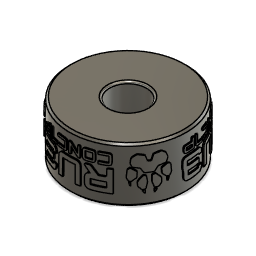
light v3 (Autodesk Fusion 360 design; units mm, degrees)
Autodesk Fusion 360 part; units mm, degrees
sketch "Esquisse1" plane through (0, 0, 0) normal (0, 1, 0) x (1, 0, 0)
  line L0 (25, 200) -> (-25, 200)
  line L1 (-25, 200) -> (-25, -200)
  line L2 (-25, -200) -> (25, -200)
  line L3 (25, -200) -> (25, 200)
  line L4 (25, 200) -> (-25, -200) construction
  line L5 (-25, 200) -> (25, -200) construction
  circle A0 centre (0, 100) radius 6.5
  circle A1 centre (0, 100) radius 4
  dimension "d1" = 50
  dimension "d2" = 400
  dimension "d3" = 13
  dimension "d4" = 8
  constraint horizontal L0
  constraint perpendicular L0 L1
  constraint parallel L0 L2
  constraint parallel L1 L3
  constraint coincident L4 origin
  constraint coincident L5 origin
  constraint concentric A0 A1
  measures "d1" distance of L1.end L2.end
  measures "d2" distance of L0.end L1.end
  measures "d3" diameter of A0
  measures "d4" diameter of A1
extrude "Extrusion1" add sketch "Esquisse1" against normal blind 6 contours L0 L1 L2 L3 makes body 1
extrude "Extrusion2" add sketch "Esquisse1" against normal blind 7 contours A0 bodies 1
fillet "Congé1" radius 3 1 edges at (-6.0601, -7, -102.3505) on bodies 1
extrude "Extrusion3" add 1 faces at (0.1619, -6, 102.1606) along direction (0, -1, 0) blind 9 and the other way blind -3 on bodies 1 bodies 1 makes body 2
extrude "Extrusion4" add sketch "Esquisse1" along normal blind -15 and the other way blind 8 contours A0 bodies 2
fillet "Congé2" radius 3 1 edges at (-6.0601, -8, -102.3505) on bodies 2
extrude "Extrusion5" add 1 faces at (0, -15, 101.3333) along direction (0, -1, 0) blind 6.5 and the other way blind -0.5 separate body on bodies 2 makes body 3
extrude "Extrusion6" add sketch "Esquisse1" along normal blind -22.5 and the other way blind 15.5 contours A0 bodies 3
fillet "Congé3" radius 3 1 edges at (-6.0601, -22.5, -102.3505) on bodies 3
extrude "Extrusion7" add sketch "Esquisse1" along normal blind 1 contours A0 bodies 1
fillet "Congé4" radius 3 1 edges at (-6.0601, 1, -97.6495) on bodies 1
extrude "Extrusion8" cut 2 faces at (-8.3333, -17.5, 200) (-8.3333, -11, 200) along direction (0, 0, -1) blind 270 on bodies 2 3 bodies 2 3
extrude "Extrusion9" add 1 faces at (-0.0996, -15, -167.9963) along direction (0, -1, 0) blind 0.25 separate body on bodies 2 makes body 4
revolve "Révolution1" add 1 faces at (-8.3333, -11, -70) angle 180 about axis through (25, -15.25, -70) along (1, 0, 0) on bodies 2 bodies 2 3 4
extrude "Extrusion10" cut 1 faces at (-0.0996, -15.25, -167.9963) along direction (0, 1, 0) blind 0.25 on bodies 2 bodies 2
sketch "Esquisse2" plane through (0, 0, 0) normal (0, -1, 0) x (1, 0, 0)
  line L0 (25, -70) -> (-25, -70)
  line L1 (-25, -70) -> (-25, -200)
  line L2 (-25, -200) -> (25, -200)
  line L3 (25, -200) -> (25, -70)
  circle A0 centre (0, -100) radius 6.5
  circle A1 centre (0, -100) radius 10
  circle A2 centre (0, -100) radius 3.5
  circle A3 centre (0, -100) radius 6.5
  line L4 (25, 200) -> (25, -200)
  line L5 (25, -200) -> (-25, -200)
  line L6 (-25, -200) -> (-25, 200)
  line L7 (-25, 200) -> (25, 200)
  dimension "d42" = 7
  constraint concentric A0 A1
  constraint concentric A1 A2
  measures "d42" diameter of A2
extrude "Extrusion11" add sketch "Esquisse2" along normal blind -1 and the other way blind 4 separate body contours A0 A3 | A1 | A2 makes body 5
fillet "Congé5" radius 2 1 edges at (-9.3233, 4, -96.3838) on bodies 5
fillet "Congé6" radius 1 1 edges at (-9.3233, 1, -96.3838) on bodies 5
extrude "Extrusion12" add sketch "Esquisse2" along normal blind 22.5 and the other way blind 1 contours A2 bodies 5
extrude "Extrusion13" add 1 faces at (1.7216, -22.5, -100.6592) along direction (0, -1, 0) blind 12 on bodies 5 bodies 5
ref_plane "Plan de construction1" through (0, 0, -100) normal (0, 0, 1) x (1, 0, 0)
sketch "Esquisse3" plane through (0, 0, -100) normal (0, 0, 1) x (1, 0, 0)
  line L0 (0, -32.5) -> (0, -22.5)
  line L1 (0, -22.5) -> (0, -22.7)
  circle A0 centre (0, -25.5) radius 1.7
  line L2 (0, -34.5) -> (-1.5, -34.5)
  line L3 (-1.5, -34.5) -> (-1.5, -32.5)
  circle A1 centre (-1.5, -32.5) radius 2
  circle A2 centre (1.5, -32.5) radius 2
  line L4 (3.5, -34.5) -> (3.5, -31.3)
  line L5 (-3.5, -34.5) -> (3.5, -34.5)
  line L6 (3.5, -34.5) -> (-3.5, -34.5)
  line L7 (-3.5, -34.5) -> (-3.5, -31.3)
  dimension "d60" = 3.4
  dimension "d65" = 1.5
  dimension "d66" = 2
  dimension "d67" = 4
  constraint vertical L0
  constraint coincident L0 L1.end
  constraint horizontal L2
  constraint perpendicular L2 L3
  constraint coincident L3.end A1.centre
  constraint symmetric L0 A1 A2
  constraint vertical L4
  constraint tangent A2 L4
  constraint coincident L4.start L5
  constraint coincident L4.start L5.end
  constraint coincident L5.start L6.end
  constraint perpendicular L6 L7
  constraint coincident L0 A0.centre
  measures "d60" diameter of A0
  measures "d65" distance of L2.start L2.end
  measures "d66" distance of L2.end L3.end
  measures "d67" diameter of A1
extrude "Extrusion14" cut sketch "Esquisse3" along normal blind 5 and the other way blind 5 contours L0 A0 | L0 A0 bodies 5
thread "Filetage2" "ISO Metric profile 7.0 M7x1 6g" major diameter 6.884 minor diameter 5.744 pitch 1 angle 60 modelled right hand crest width 0.1446 on face at (-2.0275, -19.6639, -102.8529) crest through (3.442, 1.25, -100) on bodies 5
revolve "Révolution2" cut sketch "Esquisse3" angle 360 about axis through (0, -32.5, -100) along (0, 1, 0) contours A1 L5 L6 L7 | A2 L4 L5 L6 bodies 5
sketch "Esquisse5" plane through (0, -34.5, 0) normal (0, -1, 0) x (1, 0, 0)
  circle A0 centre (0, -100) radius 1.5
  circle A1 centre (0, -100) radius 15
  circle A2 centre (0, -100) radius 3.5
  circle A3 centre (0, -100) radius 5.5
  circle A4 centre (0, -100) radius 14
  circle A5 centre (0, -100) radius 13.9
  line L0 (0, -113.9) -> (12.0378, -106.95)
  line L1 (12.0378, -106.95) -> (12.0378, -93.05)
  line L2 (12.0378, -93.05) -> (0, -86.1)
  line L3 (0, -86.1) -> (-12.0378, -93.05)
  line L4 (-12.0378, -93.05) -> (-12.0378, -106.95)
  line L5 (-12.0378, -106.95) -> (0, -113.9)
  line L6 (0, -114) -> (12.1244, -107)
  line L7 (12.1244, -107) -> (12.1244, -93)
  line L8 (12.1244, -93) -> (0, -86)
  line L9 (0, -86) -> (-12.1244, -93)
  line L10 (-12.1244, -93) -> (-12.1244, -107)
  line L11 (-12.1244, -107) -> (0, -114)
  point P0 (0, -100)
  point P1 (0, -100)
  dimension "d69" = 30
  dimension "d70" = 7
  dimension "d71" = 11
  dimension "d94" = -1
  dimension "d95" = -1.1
  constraint concentric A0 A1
  constraint concentric A1 A2
  constraint concentric A1 A3
  constraint coincident P1 P0
  constraint coincident A5 L0.start
  constraint coincident A4 L6.start
  measures "d69" diameter of A1
  measures "d70" diameter of A2
  measures "d71" diameter of A3
extrude "Extrusion16" add sketch "Esquisse5" against normal blind 7 separate body contours A2 | A3 | L0 L1 L2 L3 L4 L5 makes body 6
extrude "Extrusion19" add sketch "Esquisse5" against normal blind 7 separate body contours A0 | A1 | A2 | A3 | A4 A5 L7 | A4 A5 L8 | A5 L7 L8 | A4 A5 L6 | A5 L6 L7 | A4 A5 L9 | A5 L8 L9 | A5 L1 L7 | A5 L7 | A5 L8 | A5 L2 L8 | A5 L6 L11 | A4 A5 L11 | A5 L0 L6 | A5 L6 | A4 A5 L10 | A5 L9 L10 | A5 L9 | A5 L3 L9 | L0 L1 L2 L3 L4 L5 | A5 L10 L11 | A5 L5 L11 | A5 L11 | A5 L10 | A5 L4 L10 makes body 7
extrude "Extrusion18" add sketch "Esquisse5" along normal blind 7 contours A0 | A1 | A2 | A3 | A4 A5 L7 | A4 A5 L8 | A5 L7 L8 | A4 A5 L6 | A5 L6 L7 | A4 A5 L9 | A5 L8 L9 | A5 L1 L7 | A5 L7 | A5 L8 | A5 L2 L8 | A5 L6 L11 | A4 A5 L11 | A5 L0 L6 | A5 L6 | A4 A5 L10 | A5 L9 L10 | A5 L9 | A5 L3 L9 | L0 L1 L2 L3 L4 L5 | A5 L10 L11 | A5 L5 L11 | A5 L11 | A5 L10 | A5 L4 L10 bodies 7
chamfer "Chanfrein1" distance 0.5 angle 45 1 edges at (-13.9849, -41.5, -105.4242) on bodies 7
thread "Filetage4" "ISO Metric profile 7.0 M7x1 6H" major diameter 7.1472 minor diameter 6.0355 pitch 1 angle 60 modelled right hand crest width 0.2748 on face at (-1.3822, -29.8333, -99.4173) crest through (3.0178, -34.25, -100) on bodies 6
sketch "Esquisse8" plane through (0, -41.5, 0) normal (0, -1, 0) x (1, 0, 0)
  circle A0 centre (0, -100) radius 14.5
  line L0 (3.6323, -106.3615) -> (-0.1725, -106.3593)
  line L1 (-0.2143, -104.9499) -> (7.6688, -104.9708)
  line L2 (-0.1873, -89.7876) -> (0.9346, -89.7876)
  line L3 (-3.9773, -106.357) -> (-4.3209, -106.726)
  line L4 (-9.0437, -107.0514) -> (-9.6909, -106.1227)
  line L5 (0.9346, -89.7876) -> (1.6924, -90.8691)
  line L6 (3.9917, -98.7256) -> (1.9715, -95.3789)
  line L7 (3.1281, -92.9522) -> (3.806, -93.9537)
  line L8 (1.9715, -95.3789) -> (-0.0487, -92.0323)
  line L9 (-4.3209, -106.726) -> (-4.6645, -107.0949)
  line L10 (-8.0974, -104.9291) -> (-0.2143, -104.9499)
  line L11 (-4.1291, -98.3583) -> (-5.1879, -100.1132)
  line L12 (-6.0052, -98.5623) -> (-4.6592, -96.5217)
  line L13 (8.6765, -107.0922) -> (6.476, -107.0922)
  line L14 (4.803, -100.0724) -> (3.9917, -98.7256)
  line L15 (5.3675, -98.1557) -> (6.929, -100.5213)
  line L16 (-0.1725, -106.3593) -> (-3.9773, -106.357)
  line L17 (1.6924, -90.8691) -> (2.4502, -91.9506)
  line L18 (9.9911, -105.1511) -> (9.3338, -106.1216)
  line L19 (-7.3512, -100.603) -> (-6.0052, -98.5623)
  line L20 (3.806, -93.9537) -> (3.806, -94.8719)
  line L21 (-0.0878, -91.9667) -> (-0.127, -91.9012)
  line L22 (-0.127, -91.9012) -> (-0.1974, -91.9259)
  line L23 (7.3112, -104.2279) -> (6.8873, -103.5514)
  line L24 (2.4502, -91.9506) -> (3.1281, -92.9522)
  line L25 (-4.6645, -107.0949) -> (-6.8541, -107.0732)
  line L26 (3.806, -94.8719) -> (3.806, -95.7901)
  line L27 (-6.8541, -107.0732) -> (-9.0437, -107.0514)
  line L28 (8.46, -102.8362) -> (9.9911, -105.1511)
  line L29 (3.806, -95.7901) -> (5.3675, -98.1557)
  line L30 (-0.0487, -92.0323) -> (-0.0878, -91.9667)
  line L31 (6.476, -107.0922) -> (4.2755, -107.0922)
  line L32 (-4.1117, -94.7561) -> (-4.1117, -93.8237)
  line L33 (6.929, -100.5213) -> (8.46, -102.8362)
  line L34 (6.0639, -102.1539) -> (5.6142, -101.4192)
  line L35 (-4.1117, -95.6885) -> (-4.1117, -94.7561)
  line L36 (7.7352, -104.9044) -> (7.3112, -104.2279)
  line L37 (9.3338, -106.1216) -> (8.6765, -107.0922)
  line L38 (-5.1879, -100.1132) -> (-6.6427, -102.5212)
  line L39 (-10.3381, -105.1939) -> (-10.189, -104.9391)
  line L40 (6.8873, -103.5514) -> (6.7004, -103.2199)
  line L41 (7.702, -104.9376) -> (7.7352, -104.9044)
  line L42 (-1.669, -94.277) -> (-3.0702, -96.6033)
  line L43 (-0.1974, -91.9259) -> (-0.2678, -91.9506)
  line L44 (5.6142, -101.4192) -> (4.803, -100.0724)
  line L45 (-10.0399, -104.6843) -> (-8.6956, -102.6436)
  line L46 (-4.6592, -96.5217) -> (-4.3854, -96.1051)
  line L47 (4.2755, -107.0922) -> (3.9539, -106.7269)
  line L48 (3.9539, -106.7269) -> (3.6323, -106.3615)
  line L49 (-1.3091, -89.7876) -> (-0.1873, -89.7876)
  line L50 (7.6688, -104.9708) -> (7.702, -104.9376)
  line L51 (-3.0702, -96.6033) -> (-4.1291, -98.3583)
  line L52 (-4.3854, -96.1051) -> (-4.1117, -95.6885)
  line L53 (6.7004, -103.2199) -> (6.5135, -102.8885)
  line L54 (-2.7104, -91.8056) -> (-1.3091, -89.7876)
  line L55 (-0.2678, -91.9506) -> (-1.669, -94.277)
  line L56 (6.5135, -102.8885) -> (6.0639, -102.1539)
  line L57 (-6.6427, -102.5212) -> (-8.0974, -104.9291)
  line L58 (-8.6956, -102.6436) -> (-7.3512, -100.603)
  line L59 (-4.1117, -93.8237) -> (-2.7104, -91.8056)
  line L60 (-10.189, -104.9391) -> (-10.0399, -104.6843)
  line L61 (-9.6909, -106.1227) -> (-10.3381, -105.1939)
  line L62 (0.0438, -98.9394) -> (0.1799, -98.4652)
  line L63 (0.1799, -98.4652) -> (0.3161, -97.9909)
  line L64 (2.3261, -98.8888) -> (2.2791, -99.0929)
  line L65 (0.3615, -97.9392) -> (0.8389, -97.8251)
  line L66 (0.4669, -100.7254) -> (-0.1695, -100.7242)
  line L67 (1.398, -97.7151) -> (1.4797, -97.7192)
  line L68 (0.4669, -100.7254) -> (-0.1695, -100.7242)
  line L69 (1.7654, -97.9205) -> (2.051, -98.1218)
  line L70 (2.051, -98.1218) -> (2.1886, -98.5053)
  line L71 (2.051, -98.1218) -> (2.1886, -98.5053)
  line L72 (1.398, -97.7151) -> (1.4797, -97.7192)
  line L73 (2.3261, -98.8888) -> (2.2791, -99.0929)
  line L74 (0.3388, -97.9651) -> (0.3615, -97.9392)
  line L75 (0.7858, -103.6458) -> (0.6253, -103.8385)
  line L76 (0.8389, -97.8251) -> (1.3164, -97.7111)
  line L77 (0.4621, -103.766) -> (0.4593, -103.5007)
  line L78 (-0.604, -101.2643) -> (-0.5379, -101.7499)
  line L79 (0.4648, -104.0313) -> (0.4621, -103.766)
  line L80 (0.3615, -97.9392) -> (0.8389, -97.8251)
  line L81 (-2.2222, -101.657) -> (-2.5922, -101.957)
  line L82 (2.7983, -100.7801) -> (2.8481, -101.4264)
  line L83 (2.2791, -99.0929) -> (2.2322, -99.297)
  line L84 (-2.4384, -99.6984) -> (-2.5818, -99.4161)
  line L85 (2.1886, -98.5053) -> (2.3261, -98.8888)
  line L86 (1.8369, -101.6417) -> (1.5066, -101.3336)
  line L87 (0.1328, -101.7824) -> (0.1328, -101.2414)
  line L88 (-0.6144, -98.4472) -> (-0.4648, -98.8888)
  line L89 (0.1799, -98.4652) -> (0.3161, -97.9909)
  line L90 (0.6253, -103.8385) -> (0.4648, -104.0313)
  line L91 (0.0438, -98.9394) -> (0.1799, -98.4652)
  line L92 (-2.4384, -99.6984) -> (-2.5818, -99.4161)
  line L93 (-0.2105, -98.9141) -> (0.0438, -98.9394)
  line L94 (2.1886, -98.5053) -> (2.3261, -98.8888)
  line L95 (2.2791, -99.0929) -> (2.2322, -99.297)
  line L96 (-2.9199, -101.909) -> (-3.0739, -101.6445)
  line L97 (1.7654, -97.9205) -> (2.051, -98.1218)
  line L98 (-1.057, -101.1335) -> (-0.9314, -101.1348)
  line L99 (-0.764, -98.0056) -> (-0.6144, -98.4472)
  line L100 (-1.4182, -99.9122) -> (-1.6018, -99.8695)
  line L101 (1.4797, -97.7192) -> (1.7654, -97.9205)
  line L102 (-1.8307, -97.7061) -> (-1.3304, -97.8228)
  line L103 (-2.4722, -98.111) -> (-2.1515, -97.9085)
  line L104 (-1.4182, -99.9122) -> (-1.6018, -99.8695)
  line L105 (1.3164, -97.7111) -> (1.398, -97.7151)
  line L106 (-0.8301, -97.9395) -> (-0.797, -97.9726)
  line L107 (-0.5632, -102.6892) -> (-0.6544, -103.1429)
  line L108 (-2.6424, -102.113) -> (-2.6424, -102.4151)
  line L109 (-0.6144, -98.4472) -> (-0.4648, -98.8888)
  line L110 (1.4797, -97.7192) -> (1.7654, -97.9205)
  line L111 (0.3161, -97.9909) -> (0.3388, -97.9651)
  line L112 (-0.4648, -98.8888) -> (-0.2105, -98.9141)
  line L113 (0.3161, -97.9909) -> (0.3388, -97.9651)
  line L114 (-2.6849, -98.7835) -> (-2.6447, -98.4333)
  line L115 (1.3164, -97.7111) -> (1.398, -97.7151)
  line L116 (-0.4648, -98.8888) -> (-0.2105, -98.9141)
  line L117 (0.8389, -97.8251) -> (1.3164, -97.7111)
  line L118 (0.3388, -97.9651) -> (0.3615, -97.9392)
  line L119 (0.5989, -101.0519) -> (1.0189, -101.496)
  line L120 (-1.636, -101.8274) -> (-1.3465, -101.4804)
  line L121 (-0.797, -97.9726) -> (-0.764, -98.0056)
  line L122 (-1.8307, -97.7061) -> (-1.3304, -97.8228)
  line L123 (-0.797, -97.9726) -> (-0.764, -98.0056)
  line L124 (-2.7252, -99.1337) -> (-2.6849, -98.7835)
  line L125 (-0.8059, -100.7229) -> (-0.8957, -100.6629)
  line L126 (-2.905, -102.113) -> (-2.7737, -102.113)
  line L127 (0.8675, -100.0614) -> (0.745, -100.2178)
  line L128 (0.5487, -101.0519) -> (0.5738, -101.0519)
  line L129 (-3.1118, -100.1414) -> (-2.9434, -99.9845)
  line L130 (2.1672, -101.9498) -> (1.8369, -101.6417)
  line L131 (-1.7749, -102.4757) -> (-1.8038, -102.1539)
  line L132 (0.6226, -103.5007) -> (0.7858, -103.5007)
  line L133 (0.9899, -99.9051) -> (0.8675, -100.0614)
  line L134 (-2.7561, -101.933) -> (-2.9199, -101.909)
  line L135 (0.745, -100.2178) -> (0.606, -100.4716)
  line L136 (1.5066, -101.3336) -> (1.4727, -100.8867)
  line L137 (0.3407, -101.1466) -> (0.5487, -101.0519)
  line L138 (-2.7183, -102.6395) -> (-2.7941, -102.562)
  line L139 (2.3884, -102.1106) -> (2.2571, -102.1106)
  line L140 (2.2571, -102.1106) -> (2.2571, -102.4126)
  line L141 (2.8481, -101.4264) -> (2.7128, -101.6881)
  line L142 (-1.8354, -100.8921) -> (-1.8522, -101.3569)
  line L143 (1.4727, -100.8867) -> (1.4388, -100.4397)
  line L144 (1.2219, -102.9797) -> (1.005, -103.2641)
  line L145 (-2.247, -100.1274) -> (-1.8186, -100.4273)
  line L146 (-1.7854, -99.8268) -> (-2.1119, -99.7626)
  line L147 (2.7128, -101.6881) -> (2.5774, -101.9498)
  line L148 (1.4389, -101.94) -> (1.4389, -102.3177)
  line L149 (0.1328, -101.2414) -> (0.3407, -101.1466)
  line L150 (-1.8522, -101.3569) -> (-2.2222, -101.657)
  line L151 (-0.1695, -100.7242) -> (-0.8059, -100.7229)
  line L152 (2.0221, -99.7149) -> (1.506, -99.81)
  line L153 (-0.9987, -103.3374) -> (-1.2228, -103.3374)
  line L154 (0.606, -100.4716) -> (0.4669, -100.7254)
  line L155 (2.6038, -100.0241) -> (2.7484, -100.1338)
  line L156 (2.4088, -102.5596) -> (2.4642, -102.3351)
  line L157 (-1.2018, -100.2576) -> (-1.4182, -99.9122)
  line L158 (-1.8186, -100.4273) -> (-1.8354, -100.8921)
  line L159 (1.4389, -102.3177) -> (1.4389, -102.6953)
  line L160 (-2.8496, -102.3375) -> (-2.905, -102.113)
  line L161 (-2.6424, -102.7171) -> (-2.7183, -102.6395)
  line L162 (2.2571, -102.7146) -> (2.3329, -102.6371)
  line L163 (0.8675, -100.0614) -> (0.745, -100.2178)
  line L164 (1.8461, -100.1744) -> (2.2534, -99.9092)
  line L165 (2.7484, -100.1338) -> (2.7983, -100.7801)
  line L166 (-0.765, -103.4191) -> (-0.765, -103.7047)
  line L167 (-1.0035, -103.495) -> (-0.8875, -103.4216)
  line L168 (-2.7749, -99.8275) -> (-2.7252, -99.8275)
  line L169 (-0.7146, -103.2402) -> (-0.7747, -103.3374)
  line L170 (-3.2279, -101.38) -> (-3.1699, -100.7607)
  line L171 (-0.9812, -103.7794) -> (-1.1195, -103.5684)
  line L172 (-0.7747, -103.3374) -> (-0.9987, -103.3374)
  line L173 (-1.7854, -99.8268) -> (-2.1119, -99.7626)
  line L174 (0.4458, -103.215) -> (0.2893, -102.7692)
  line L175 (2.0221, -99.7149) -> (1.506, -99.81)
  line L176 (-1.2228, -103.3374) -> (-1.4844, -103.0675)
  line L177 (0.2893, -102.7692) -> (0.1328, -102.3234)
  line L178 (-2.7252, -99.8275) -> (-2.6755, -99.8275)
  line L179 (2.4642, -102.3351) -> (2.5197, -102.1106)
  line L180 (-0.8263, -103.4203) -> (-0.765, -103.4191)
  line L181 (0.7858, -103.5733) -> (0.7858, -103.6458)
  line L182 (-1.6018, -99.8695) -> (-1.7854, -99.8268)
  line L183 (1.005, -103.2641) -> (0.7254, -103.2396)
  line L184 (0.4593, -103.5007) -> (0.6226, -103.5007)
  line L185 (-0.6544, -103.1429) -> (-0.7146, -103.2402)
  line L186 (-1.1195, -103.5684) -> (-1.0035, -103.495)
  line L187 (2.3563, -99.9118) -> (2.4592, -99.9143)
  line L188 (-3.0739, -101.6445) -> (-3.2279, -101.38)
  line L189 (-0.765, -103.7047) -> (-0.765, -103.9904)
  line L190 (-0.804, -103.9904) -> (-0.8429, -103.9904)
  line L191 (-0.765, -103.9904) -> (-0.804, -103.9904)
  line L192 (-0.8875, -103.4216) -> (-0.8263, -103.4203)
  line L193 (-0.8429, -103.9904) -> (-0.9812, -103.7794)
  line L194 (2.5774, -101.9498) -> (2.3723, -101.9498)
  line L195 (0.7858, -103.5007) -> (0.7858, -103.5733)
  line L196 (-2.1119, -99.7626) -> (-2.4384, -99.6984)
  line L197 (2.2571, -102.4126) -> (2.2571, -102.7146)
  line L198 (0.745, -100.2178) -> (0.606, -100.4716)
  line L199 (-0.8957, -100.6629) -> (-0.9855, -100.603)
  line L200 (-1.3465, -101.4804) -> (-1.057, -101.1335)
  line L201 (0.606, -100.4716) -> (0.4669, -100.7254)
  line L202 (1.4388, -100.4397) -> (1.8461, -100.1744)
  line L203 (-2.5818, -99.4161) -> (-2.7252, -99.1337)
  line L204 (-0.9855, -100.603) -> (-1.2018, -100.2576)
  line L205 (-1.6018, -99.8695) -> (-1.7854, -99.8268)
  line L206 (-2.1515, -97.9085) -> (-1.8307, -97.7061)
  line L207 (2.4592, -99.9143) -> (2.6038, -100.0241)
  line L208 (-2.6447, -98.4333) -> (-2.5584, -98.2721)
  line L209 (2.3723, -101.9498) -> (2.1672, -101.9498)
  line L210 (-2.1119, -99.7626) -> (-2.4384, -99.6984)
  line L211 (-0.8059, -100.7229) -> (-0.8957, -100.6629)
  line L212 (-2.5584, -98.2721) -> (-2.4722, -98.111)
  line L213 (0.9899, -99.9051) -> (0.8675, -100.0614)
  line L214 (1.4389, -102.6953) -> (1.2219, -102.9797)
  line L215 (0.5738, -101.0519) -> (0.5989, -101.0519)
  line L216 (2.1271, -99.5059) -> (2.0221, -99.7149)
  line L217 (-2.7941, -102.562) -> (-2.8496, -102.3375)
  line L218 (-2.5818, -99.4161) -> (-2.7252, -99.1337)
  line L219 (-2.5922, -101.957) -> (-2.7561, -101.933)
  line L220 (-0.5379, -101.7499) -> (-0.4719, -102.2355)
  line L221 (-3.1699, -100.7607) -> (-3.1118, -100.1414)
  line L222 (2.3329, -102.6371) -> (2.4088, -102.5596)
  line L223 (2.2322, -99.297) -> (2.1271, -99.5059)
  line L224 (-0.1695, -100.7242) -> (-0.8059, -100.7229)
  line L225 (-2.6447, -98.4333) -> (-2.5584, -98.2721)
  line L226 (-1.8038, -102.1539) -> (-1.7199, -101.9906)
  line L227 (-1.2018, -100.2576) -> (-1.4182, -99.9122)
  line L228 (-0.764, -98.0056) -> (-0.6144, -98.4472)
  line L229 (-2.6849, -98.7835) -> (-2.6447, -98.4333)
  line L230 (-0.2105, -98.9141) -> (0.0438, -98.9394)
  line L231 (1.0189, -101.496) -> (1.4389, -101.94)
  line L232 (2.2322, -99.297) -> (2.1271, -99.5059)
  line L233 (-2.6424, -102.4151) -> (-2.6424, -102.7171)
  line L234 (-2.4722, -98.111) -> (-2.1515, -97.9085)
  line L235 (-2.7737, -102.113) -> (-2.6424, -102.113)
  line L236 (-0.7049, -101.2002) -> (-0.604, -101.2643)
  line L237 (-1.3304, -97.8228) -> (-0.8301, -97.9395)
  line L238 (-2.5584, -98.2721) -> (-2.4722, -98.111)
  line L239 (0.1328, -102.3234) -> (0.1328, -101.7824)
  line L240 (-0.8301, -97.9395) -> (-0.797, -97.9726)
  line L241 (-2.9434, -99.9845) -> (-2.7749, -99.8275)
  line L242 (2.1271, -99.5059) -> (2.0221, -99.7149)
  line L243 (-1.3304, -97.8228) -> (-0.8301, -97.9395)
  line L244 (-0.9314, -101.1348) -> (-0.8059, -101.136)
  line L245 (-0.8059, -101.136) -> (-0.7049, -101.2002)
  line L246 (2.2534, -99.9092) -> (2.3563, -99.9118)
  line L247 (-1.746, -102.7976) -> (-1.7749, -102.4757)
  line L248 (1.506, -99.81) -> (0.9899, -99.9051)
  line L249 (-0.9855, -100.603) -> (-1.2018, -100.2576)
  line L250 (-0.4719, -102.2355) -> (-0.5632, -102.6892)
  line L251 (0.7254, -103.2396) -> (0.4458, -103.215)
  line L252 (-1.7199, -101.9906) -> (-1.636, -101.8274)
  line L253 (2.5197, -102.1106) -> (2.3884, -102.1106)
  line L254 (-0.8957, -100.6629) -> (-0.9855, -100.603)
  line L255 (-2.7252, -99.1337) -> (-2.6849, -98.7835)
  line L256 (-2.6755, -99.8275) -> (-2.247, -100.1274)
  line L257 (-1.4844, -103.0675) -> (-1.746, -102.7976)
  line L258 (1.506, -99.81) -> (0.9899, -99.9051)
  line L259 (-2.1515, -97.9085) -> (-1.8307, -97.7061)
  circle A1 centre (0, -100) radius 14.5
emboss "Gravure en relief2" depth -0.4 profiles "Esquisse8" section 1 contours L0 L2 L3 L4 L5 L7 L9 L12 L13 L15 L16 L17 L18 L19 L20 L24 L25 L26 L27 L28 L29 L31 L32 L33 L35 L37 L39 L45 L46 L47 L48 L49 L52 L54 L58 L59 L60 L61 | L62 L63 L64 L65 L66 L67 L68 L69 L70 L71 L72 L73 L74 L76 L80 L83 L84 L85 L88 L89 L91 L92 L93 L94 L95 L97 L99 L100 L101 L102 L103 L104 L105 L106 L109 L110 L111 L112 L113 L114 L115 L116 L117 L118 L121 L122 L123 L124 L125 L127 L133 L135 L146 L151 L152 L154 L157 L163 L173 L175 L182 L196 L198 L199 L201 L203 L204 L205 L206 L208 L210 L211 L212 L213 L216 L218 L223 L224 L225 L227 L228 L229 L230 L232 L234 L237 L238 L240 L242 L243 L248 L249 L254 L255 L258 L259 | L75 L77 L79 L90 L132 L181 L184 L195 | L78 L98 L107 L120 L131 L153 L169 L172 L176 L185 L200 L220 L226 L236 L244 L245 L247 L250 L252 L257 | L81 L96 L129 L134 L142 L145 L150 L158 L168 L170 L178 L188 L219 L221 L241 L256 | L82 L86 L130 L136 L141 L143 L147 L155 L164 L165 L187 L194 L202 L207 L209 L246 | L87 L119 L128 L137 L144 L148 L149 L159 L174 L177 L183 L214 L215 L231 L239 L251 | L108 L126 L138 L160 L161 L217 L233 L235 | L139 L140 L156 L162 L179 L197 L222 L253 | L166 L167 L171 L180 L186 L189 L190 L191 L192 L193 onto face at (9.3024, -41.5, -103.9344) on bodies 7 bodies 7
sketch "Esquisse9" plane through (0, 0, 0) normal (0, 0, 1) x (1, 0, 0)
  line L0 (18.0757, -34.7535) -> (18.0282, -34.1284)
  line L1 (11.4541, -34.8184) -> (11.5353, -33.9522)
  line L2 (13.4251, -33.4859) -> (13.4016, -34.136)
  line L3 (14.4903, -34.4736) -> (14.6659, -34.4754)
  line L4 (19.8821, -33.9793) -> (19.9518, -34.8832)
  line L5 (-7.8492, -34.7645) -> (-7.8492, -35.2972)
  spline S0 degree 3 poles (7.4266, -29.6855) (8.5421, -29.6855) (8.5702, -29.6892) (8.7408, -29.8598) knots 0 0 0 0 1 1 1 1
  line L6 (-7.5083, -30.5933) -> (-6.6061, -30.5734)
  line L7 (-6.2864, -34.2317) -> (-7.8492, -34.2317)
  line L8 (1.1658, -31.2181) -> (0.6395, -30.5841)
  line L9 (0.0357, -32.3934) -> (0.0357, -31.0394)
  line L10 (-8.1195, -31.4791) -> (-8.1411, -31.8165)
  line L11 (-6.6061, -30.5734) -> (-6.5849, -30.1294)
  line L12 (3.7296, -31.0351) -> (3.7296, -31.8165)
  spline S1 degree 3 poles (-8.5303, -32.15) (-8.7648, -31.8771) (-8.7799, -31.0828) (-8.556, -30.7982) knots 0 0 0 0 1 1 1 1
  line L13 (-5.2564, -29.6855) -> (-5.0078, -29.6855)
  line L14 (-3.0898, -32.1054) -> (-3.0898, -31.8165)
  spline S2 degree 3 poles (5.7352, -29.928) (5.7639, -29.9704) (5.7879, -30.4717) (5.7885, -31.0419) knots 0 0 0 0 1 1 1 1
  line L15 (-8.359, -32.3493) -> (-8.5303, -32.15)
  line L16 (-6.2815, -29.6855) -> (-5.9991, -29.6855)
  line L17 (0.604, -31.4667) -> (0.5685, -32.3493)
  line L18 (-1.6002, -38.5648) -> (-2.1701, -38.5648)
  line L19 (-4.5105, -35.8655) -> (-4.5105, -36.4338)
  spline S3 degree 3 poles (-4.2168, -32.3848) (-5.0338, -32.3848) (-5.1505, -32.3692) (-5.3179, -32.2376) knots 0 0 0 0 1 1 1 1
  line L20 (-5.505, -29.6855) -> (-5.2564, -29.6855)
  line L21 (5.2924, -31.0351) -> (5.2924, -30.2537)
  line L22 (8.3469, -31.8165) -> (8.3469, -31.0351)
  spline S4 degree 3 poles (5.7885, -31.0419) (5.7899, -32.3794) (5.824, -32.34) (4.6394, -32.3731) knots 0 0 0 0 1 1 1 1
  line L23 (7.3169, -31.8165) -> (8.3469, -31.8165)
  line L24 (-8.1411, -31.8165) -> (-7.3558, -31.8165)
  line L25 (-7.8492, -35.2972) -> (-6.1799, -35.2972)
  line L26 (-2.7401, -38.5648) -> (-2.7196, -36.1903)
  line L27 (-4.1554, -37.0021) -> (-3.5871, -37.0021)
  line L28 (-7.6361, -36.931) -> (-7.6361, -37.4283)
  line L29 (-3.981, -38.2839) -> (-4.2341, -38.5293)
  line L30 (-4.7236, -37.4283) -> (-4.7236, -37.2152)
  spline S5 degree 3 poles (8.7408, -29.8598) (8.9093, -30.0283) (8.9151, -30.067) (8.9129, -31.0141) knots 0 0 0 0 1 1 1 1
  line L31 (0.3021, -32.3713) -> (0.0357, -32.3934)
  spline S6 degree 3 poles (-8.556, -30.7982) (-8.4146, -30.6183) (-8.385, -30.6126) (-7.5083, -30.5933) knots 0 0 0 0 1 1 1 1
  line L32 (6.2869, -31.8165) -> (7.3169, -31.8165)
  line L33 (9.1283, -38.5648) -> (6.7591, -38.5648)
  spline S7 degree 3 poles (-0.6487, -29.8327) (-0.4616, -29.9799) (-0.4615, -29.9802) (-0.4615, -31.0293) knots 0 0 0 0 1 1 1 1
  line L34 (-3.0898, -29.9696) -> (-3.0898, -29.6855)
  line L35 (-3.3029, -32.1007) -> (-3.3029, -32.3848)
  line L36 (-7.6361, -37.4283) -> (-6.1799, -37.4283)
  line L37 (-7.3342, -31.1215) -> (-8.0978, -31.1417)
  line L38 (-6.5638, -29.6855) -> (-6.2815, -29.6855)
  spline S8 degree 3 poles (-8.7725, -36.9242) (-8.7727, -36.2516) (-8.8006, -35.9736) (-8.8849, -35.8045) knots 0 0 0 0 1 1 1 1
  line L39 (-3.5871, -37.0021) -> (-3.5875, -37.2685)
  line L40 (-2.1701, -38.5648) -> (-2.7401, -38.5648)
  spline S9 degree 3 poles (-8.2584, -38.425) (-8.6945, -38.1556) (-8.7722, -37.929) (-8.7725, -36.9242) knots 0 0 0 0 1 1 1 1
  spline S10 degree 3 poles (-8.8032, -33.544) (-8.4911, -33.1191) (-8.3574, -33.0954) (-6.2792, -33.0952) knots 0 0 0 0 1 1 1 1
  line L41 (6.3579, -36.0786) -> (4.7951, -36.0786)
  line L42 (-5.0078, -29.6855) -> (-5.0078, -30.751)
  line L43 (-3.0898, -30.2537) -> (-3.0898, -29.9696)
  line L44 (-6.5849, -30.1294) -> (-6.5638, -29.6855)
  line L45 (6.3605, -34.942) -> (7.1073, -34.942)
  line L46 (-6.5706, -31.4589) -> (-6.5706, -31.1014)
  line L47 (-5.3179, -32.2376) -> (-5.505, -32.0903)
  line L48 (5.2924, -31.8165) -> (5.2924, -31.0351)
  line L49 (2.1512, -30.5897) -> (2.171, -29.6855)
  line L50 (-1.5814, -36.416) -> (-1.6002, -38.5648)
  spline S11 degree 3 poles (2.4298, -32.3848) (2.1652, -32.3848) (2.0329, -32.2627) (1.1658, -31.2181) knots 0 0 0 0 1 1 1 1
  line L51 (7.9562, -33.1306) -> (8.5422, -33.11)
  line L52 (-7.1984, -32.3493) -> (-8.359, -32.3493)
  spline S12 degree 3 poles (7.1073, -34.942) (7.6895, -34.942) (7.8627, -34.9196) (7.8931, -34.8404) knots 0 0 0 0 1 1 1 1
  line L53 (5.2924, -30.2537) -> (4.511, -30.2537)
  line L54 (4.7951, -37.4283) -> (6.3579, -37.4283)
  line L55 (-5.505, -32.0903) -> (-5.505, -30.8879)
  line L56 (6.2869, -32.1007) -> (6.2869, -31.8165)
  spline S13 degree 3 poles (5.541, -29.7703) (5.6191, -29.8147) (5.7065, -29.8856) (5.7352, -29.928) knots 0 0 0 0 1 1 1 1
  line L57 (-6.0185, -31.0174) -> (-6.0378, -32.3493)
  line L58 (-3.0898, -32.3944) -> (-3.0898, -32.1054)
  line L59 (6.2869, -29.9696) -> (6.2869, -29.6855)
  line L60 (0.5685, -32.3493) -> (0.3021, -32.3713)
  line L61 (6.2869, -30.2537) -> (6.2869, -29.9696)
  spline S14 degree 3 poles (0.3144, -29.6855) (0.5837, -29.6855) (0.6188, -29.7158) (1.3622, -30.5897) knots 0 0 0 0 1 1 1 1
  spline S15 degree 3 poles (8.9129, -31.0141) (8.9097, -32.3864) (8.9115, -32.3848) (7.3571, -32.3848) knots 0 0 0 0 1 1 1 1
  spline S16 degree 3 poles (-8.9737, -34.662) (-8.9535, -33.868) (-8.9305, -33.7173) (-8.8032, -33.544) knots 0 0 0 0 1 1 1 1
  line L62 (7.3169, -30.2537) -> (6.2869, -30.2537)
  line L63 (7.3571, -32.3848) -> (6.2869, -32.3848)
  line L64 (0.0357, -31.0394) -> (0.0357, -29.6855)
  line L65 (8.3469, -30.2537) -> (7.3169, -30.2537)
  line L66 (6.2869, -32.3848) -> (6.2869, -32.1007)
  line L67 (0.0357, -29.6855) -> (0.3144, -29.6855)
  line L68 (8.3469, -31.0351) -> (8.3469, -30.2537)
  line L69 (0.6395, -30.5841) -> (0.604, -31.4667)
  line L70 (-0.9588, -31.0351) -> (-0.9588, -30.2537)
  line L71 (18.5504, -33.1323) -> (19.12, -32.7612)
  line L72 (7.9441, -33.9347) -> (7.9562, -33.1306)
  spline S17 degree 3 poles (7.9295, -36.8955) (7.9295, -36.6806) (7.9275, -36.4089) (7.9251, -36.2917) knots 0 0 0 0 1 1 1 1
  line L73 (14.8539, -30.0528) -> (14.9001, -30.099)
  line L74 (16.3732, -36.7612) -> (16.1543, -36.1377)
  line L75 (-3.3029, -32.3848) -> (-4.2168, -32.3848)
  spline S18 degree 3 poles (6.3579, -37.4283) (7.3494, -37.4283) (7.9223, -37.4023) (7.9251, -37.3572) knots 0 0 0 0 1 1 1 1
  line L76 (16.8161, -33.5478) -> (16.6216, -33.9028)
  line L77 (19.3374, -36.468) -> (19.4149, -36.1541)
  line L78 (17.0696, -37.9849) -> (16.8431, -38.2568)
  line L79 (12.3578, -32.0716) -> (12.1572, -31.6767)
  line L80 (-2.0243, -30.2537) -> (-3.0898, -30.2537)
  line L81 (7.9207, -36.0786) -> (6.3579, -36.0786)
  line L82 (19.2217, -31.3343) -> (19.1561, -31.6197)
  spline S19 degree 3 poles (4.4545, -29.6876) (5.0236, -29.6889) (5.4554, -29.7218) (5.541, -29.7703) knots 0 0 0 0 1 1 1 1
  line L83 (17.0105, -33.1929) -> (16.8161, -33.5478)
  line L84 (19.1252, -35.8401) -> (19.1252, -36.2625)
  line L85 (-3.5672, -34.5869) -> (-4.1454, -34.5869)
  line L86 (3.7296, -31.8165) -> (4.511, -31.8165)
  line L87 (14.1079, -29.8434) -> (14.8076, -30.0066)
  line L88 (18.9435, -32.1973) -> (18.7966, -32.4895)
  line L89 (17.8096, -29.6871) -> (17.9238, -29.6928)
  line L90 (16.592, -37.3847) -> (16.3732, -36.7612)
  line L91 (13.4716, -32.6461) -> (13.015, -32.5563)
  line L92 (13.7284, -32.7058) -> (13.4716, -32.6461)
  line L93 (12.5111, -30.2464) -> (12.9596, -29.9633)
  line L94 (19.1252, -36.2625) -> (19.1252, -36.6849)
  line L95 (19.0294, -30.7979) -> (19.2217, -31.3343)
  line L96 (-0.9588, -31.8165) -> (-0.9588, -31.0351)
  line L97 (19.8124, -33.0754) -> (19.8821, -33.9793)
  line L98 (-3.3029, -31.8165) -> (-3.3029, -32.1007)
  spline S20 degree 3 poles (7.9251, -37.3572) (7.9275, -37.3182) (7.9295, -37.1104) (7.9295, -36.8955) knots 0 0 0 0 1 1 1 1
  line L99 (-4.7236, -34.2317) -> (-6.2864, -34.2317)
  line L100 (19.0904, -31.905) -> (18.9435, -32.1973)
  spline S21 degree 3 poles (-1.9628, -29.6855) (-0.9303, -29.6855) (-0.8202, -29.6978) (-0.6487, -29.8327) knots 0 0 0 0 1 1 1 1
  line L101 (17.9238, -29.6928) -> (18.038, -29.6985)
  line L102 (19.1252, -36.6849) -> (19.2313, -36.5765)
  line L103 (5.5985, -34.0186) -> (6.3605, -34.942)
  line L104 (14.7159, -33.8155) -> (14.5902, -33.7316)
  line L105 (12.5583, -32.4665) -> (12.3578, -32.0716)
  line L106 (-3.6089, -34.1826) -> (-3.5672, -34.5869)
  line L107 (-6.1799, -37.4283) -> (-4.7236, -37.4283)
  line L108 (-4.2341, -38.5293) -> (-6.1305, -38.5487)
  line L109 (11.5353, -33.9522) -> (11.6165, -33.0861)
  line L110 (19.6101, -32.922) -> (19.8124, -33.0754)
  line L111 (16.2202, -30.7418) -> (16.4106, -30.0785)
  line L112 (-3.0898, -31.8165) -> (-2.0243, -31.8165)
  spline S22 degree 3 poles (-4.1546, -33.255) (-3.7949, -33.4998) (-3.6548, -33.738) (-3.6089, -34.1826) knots 0 0 0 0 1 1 1 1
  line L113 (12.1572, -32.6471) -> (12.2268, -32.6471)
  line L114 (13.015, -32.5563) -> (12.5583, -32.4665)
  line L115 (-6.0378, -32.3493) -> (-7.1984, -32.3493)
  spline S23 degree 3 poles (3.3016, -32.1699) (3.1752, -32.0435) (3.1613, -31.9306) (3.1613, -31.0319) knots 0 0 0 0 1 1 1 1
  line L116 (18.4375, -29.98) -> (18.8371, -30.2615)
  line L117 (19.2313, -36.5765) -> (19.3374, -36.468)
  spline S24 degree 3 poles (3.1613, -31.0319) (3.1613, -30.0673) (3.1671, -30.0284) (3.3357, -29.8598) knots 0 0 0 0 1 1 1 1
  line L118 (-3.0898, -29.6855) -> (-1.9628, -29.6855)
  line L119 (16.8431, -38.2568) -> (16.6186, -38.5263)
  line L120 (16.0298, -31.405) -> (16.2202, -30.7418)
  line L121 (-7.3558, -31.8165) -> (-6.5706, -31.8165)
  line L122 (16.6186, -38.5263) -> (16.6148, -38.1552)
  line L123 (17.9809, -36.6579) -> (17.6775, -37.0556)
  spline S25 degree 3 poles (-2.7196, -36.1903) (-2.6999, -33.9089) (-2.6933, -33.8078) (-2.5505, -33.6152) knots 0 0 0 0 1 1 1 1
  line L124 (-4.7236, -37.0021) -> (-4.1554, -37.0021)
  line L125 (17.6775, -37.0556) -> (17.3741, -37.4534)
  line L126 (17.1419, -29.8466) -> (17.8096, -29.6871)
  line L127 (3.7296, -30.2537) -> (3.7296, -31.0351)
  line L128 (17.3741, -37.4534) -> (16.9831, -37.419)
  line L129 (-8.0978, -31.1417) -> (-8.1195, -31.4791)
  line L130 (9.1283, -35.8271) -> (9.1283, -38.5648)
  line L131 (17.0676, -37.8857) -> (17.0696, -37.9849)
  line L132 (-4.1554, -31.8165) -> (-3.3029, -31.8165)
  line L133 (16.4423, -30.0423) -> (16.4741, -30.0061)
  line L134 (19.12, -32.7612) -> (19.2639, -32.7649)
  spline S26 degree 3 poles (3.3357, -29.8598) (3.5035, -29.6919) (3.545, -29.6855) (4.4545, -29.6876) knots 0 0 0 0 1 1 1 1
  line L135 (-5.9991, -29.6855) -> (-6.0185, -31.0174)
  spline S27 degree 3 poles (7.8931, -34.8404) (7.9145, -34.7845) (7.9375, -34.3769) (7.9441, -33.9347) knots 0 0 0 0 1 1 1 1
  line L136 (17.353, -32.7556) -> (17.1818, -32.9742)
  line L137 (2.171, -29.6855) -> (2.4175, -29.6855)
  line L138 (-5.505, -30.8879) -> (-5.505, -29.6855)
  line L139 (-7.8492, -34.2317) -> (-7.8492, -34.7645)
  line L140 (2.664, -32.3848) -> (2.4298, -32.3848)
  line L141 (16.6148, -38.1552) -> (16.611, -37.7842)
  line L142 (16.6216, -33.9028) -> (15.7316, -33.9011)
  line L143 (-1.5626, -34.2672) -> (-1.5814, -36.416)
  line L144 (16.611, -37.7842) -> (16.8393, -37.7842)
  line L145 (-1.925, -32.3718) -> (-3.0898, -32.3944)
  line L146 (17.9808, -33.5033) -> (18.5504, -33.1323)
  line L147 (16.9831, -37.419) -> (16.592, -37.3847)
  line L148 (-7.6361, -36.4338) -> (-7.6361, -36.931)
  spline S28 degree 3 poles (-0.4615, -31.0293) (-0.4615, -32.4182) (-0.3783, -32.3419) (-1.925, -32.3718) knots 0 0 0 0 1 1 1 1
  line L149 (-4.7236, -37.2152) -> (-4.7236, -37.0021)
  line L150 (-6.0733, -36.4338) -> (-7.6361, -36.4338)
  spline S29 degree 3 poles (-8.8849, -35.8045) (-8.974, -35.6259) (-8.9923, -35.391) (-8.9737, -34.662) knots 0 0 0 0 1 1 1 1
  spline S30 degree 3 poles (-6.1305, -38.5487) (-7.9254, -38.5669) (-8.0392, -38.5603) (-8.2584, -38.425) knots 0 0 0 0 1 1 1 1
  line L151 (9.1283, -33.0894) -> (9.1283, -35.8271)
  line L152 (-0.9588, -30.2537) -> (-2.0243, -30.2537)
  line L153 (16.8393, -37.7842) -> (17.0676, -37.7842)
  line L154 (6.2869, -29.6855) -> (7.4266, -29.6855)
  line L155 (16.4106, -30.0785) -> (16.4423, -30.0423)
  line L156 (8.5422, -33.11) -> (9.1283, -33.0894)
  line L157 (-6.5706, -31.8165) -> (-6.5706, -31.4589)
  line L158 (17.0676, -37.7842) -> (17.0676, -37.8857)
  line L159 (4.8365, -33.0951) -> (5.5985, -34.0186)
  line L160 (-6.5706, -31.1014) -> (-7.3342, -31.1215)
  spline S31 degree 3 poles (-3.5875, -37.2685) (-3.5882, -37.7033) (-3.7121, -38.0231) (-3.981, -38.2839) knots 0 0 0 0 1 1 1 1
  line L161 (18.0748, -32.6226) -> (17.353, -32.7556)
  line L162 (19.2639, -32.7649) -> (19.4079, -32.7685)
  line L163 (7.9251, -36.2917) -> (7.9207, -36.0786)
  line L164 (19.1561, -31.6197) -> (19.0904, -31.905)
  line L165 (2.1313, -31.4939) -> (2.1512, -30.5897)
  line L166 (-5.0078, -30.751) -> (-5.0078, -31.8165)
  line L167 (4.511, -31.8165) -> (5.2924, -31.8165)
  line L168 (2.664, -29.6855) -> (2.664, -31.0351)
  line L169 (13.4016, -34.136) -> (13.3781, -34.786)
  line L170 (14.0854, -34.9588) -> (14.4903, -34.4736)
  line L171 (14.9827, -34.5668) -> (15.1239, -34.6565)
  line L172 (11.9057, -35.8435) -> (12.0893, -35.8435)
  line L173 (13.5631, -35.6723) -> (13.6805, -35.444)
  line L174 (13.3781, -34.786) -> (12.8606, -35.2057)
  line L175 (11.6695, -35.1882) -> (11.4541, -34.8184)
  line L176 (11.9832, -36.1575) -> (11.9057, -35.8435)
  spline S32 degree 3 poles (3.5985, -36.9408) (3.5844, -36.421) (3.6073, -35.9137) (3.6525, -35.746) knots 0 0 0 0 1 1 1 1
  line L177 (2.1668, -38.5648) -> (1.5985, -38.5648)
  line L178 (4.7951, -36.0786) -> (4.7951, -36.7534)
  line L179 (12.114, -35.5917) -> (11.8849, -35.5581)
  line L180 (15.1239, -34.6565) -> (15.2162, -35.3356)
  spline S33 degree 3 poles (-0.007, -33.0952) (1.6841, -33.0953) (1.9482, -33.1104) (2.1654, -33.2195) knots 0 0 0 0 1 1 1 1
  spline S34 degree 3 poles (2.5738, -33.5851) (2.7334, -33.824) (2.7351, -33.8508) (2.7351, -36.1957) knots 0 0 0 0 1 1 1 1
  spline S35 degree 3 poles (2.1654, -33.2195) (2.3013, -33.2879) (2.4851, -33.4524) (2.5738, -33.5851) knots 0 0 0 0 1 1 1 1
  line L181 (15.2162, -35.3356) -> (15.3086, -36.0148)
  line L182 (14.6659, -34.4754) -> (14.8415, -34.4771)
  line L183 (1.5985, -38.5648) -> (1.5985, -36.3969)
  line L184 (12.3431, -35.6253) -> (12.114, -35.5917)
  line L185 (11.8849, -35.5581) -> (11.6695, -35.1882)
  line L186 (12.8606, -35.2057) -> (12.3431, -35.6253)
  line L187 (14.8415, -34.4771) -> (14.9827, -34.5668)
  line L188 (16.7359, -34.3595) -> (16.771, -34.3595)
  line L189 (-5.0078, -31.8165) -> (-4.1554, -31.8165)
  line L190 (-4.5105, -35.2972) -> (-4.5105, -35.8655)
  line L191 (19.4925, -35.8401) -> (19.3088, -35.8401)
  line L192 (13.9852, -32.7656) -> (13.7284, -32.7058)
  line L193 (14.8415, -33.8993) -> (14.7159, -33.8155)
  line L194 (2.4175, -29.6855) -> (2.664, -29.6855)
  line L195 (14.8986, -38.4692) -> (14.8441, -38.4692)
  line L196 (14.5718, -37.5559) -> (14.2584, -37.5559)
  line L197 (12.1572, -31.6767) -> (12.2135, -31.1869)
  line L198 (19.4079, -32.7685) -> (19.6101, -32.922)
  line L199 (19.7625, -35.2492) -> (19.5732, -35.6152)
  line L200 (14.4029, -37.8789) -> (14.5651, -37.7762)
  line L201 (18.0282, -34.1284) -> (17.9808, -33.5033)
  line L202 (18.038, -29.6985) -> (18.4375, -29.98)
  spline S36 degree 3 poles (3.6525, -35.746) (3.7518, -35.3772) (4.2101, -34.942) (4.4993, -34.942) knots 0 0 0 0 1 1 1 1
  line L203 (11.6165, -33.0861) -> (11.8521, -32.8666)
  line L204 (4.511, -30.2537) -> (3.7296, -30.2537)
  line L205 (19.4149, -36.1541) -> (19.4925, -35.8401)
  line L206 (13.4081, -29.6801) -> (14.1079, -29.8434)
  line L207 (1.3622, -30.5897) -> (2.1313, -31.4939)
  line L208 (14.8986, -38.0696) -> (14.8986, -38.4692)
  line L209 (18.9995, -35.6152) -> (18.5376, -35.1843)
  line L210 (2.664, -31.0351) -> (2.664, -32.3848)
  line L211 (17.1818, -32.9742) -> (17.0105, -33.1929)
  line L212 (12.0877, -32.6471) -> (12.1572, -32.6471)
  line L213 (-2.0243, -31.8165) -> (-0.9588, -31.8165)
  line L214 (12.9596, -29.9633) -> (13.4081, -29.6801)
  line L215 (14.8986, -37.6701) -> (14.8986, -38.0696)
  line L216 (14.7273, -37.6736) -> (14.813, -37.6718)
  line L217 (19.2864, -35.6152) -> (18.9995, -35.6152)
  line L218 (-4.7236, -34.4093) -> (-4.7236, -34.2317)
  line L219 (12.8259, -33.0665) -> (13.4251, -33.4859)
  line L220 (18.8371, -30.2615) -> (19.0294, -30.7979)
  line L221 (14.2877, -33.2486) -> (13.9852, -32.7656)
  line L222 (14.5651, -37.7762) -> (14.7273, -37.6736)
  line L223 (19.9518, -34.8832) -> (19.7625, -35.2492)
  line L224 (18.5376, -35.1843) -> (18.0757, -34.7535)
  line L225 (4.212, -33.0951) -> (4.8365, -33.0951)
  spline S37 degree 3 poles (-2.5505, -33.6152) (-2.4688, -33.505) (-2.2962, -33.3429) (-2.1671, -33.255) knots 0 0 0 0 1 1 1 1
  line L226 (18.7966, -32.4895) -> (18.0748, -32.6226)
  line L227 (12.2729, -36.2659) -> (12.2729, -36.6883)
  line L228 (16.771, -34.3595) -> (16.8062, -34.3595)
  line L229 (4.7951, -36.7534) -> (4.7951, -37.4283)
  line L230 (15.1093, -30.7166) -> (15.3185, -31.3343)
  spline S38 degree 3 poles (-4.1454, -34.5869) (-4.7148, -34.5869) (-4.7236, -34.5842) (-4.7236, -34.4093) knots 0 0 0 0 1 1 1 1
  line L231 (13.8925, -37.1784) -> (13.5266, -36.8009)
  line L232 (17.9809, -35.6015) -> (17.9809, -36.1297)
  line L233 (14.5902, -33.7316) -> (14.2877, -33.2486)
  line L234 (15.0533, -37.2838) -> (14.9692, -37.4199)
  line L235 (13.4862, -36.3507) -> (13.4458, -35.9006)
  spline S39 degree 3 poles (4.1551, -38.405) (3.6796, -38.0814) (3.6256, -37.9393) (3.5985, -36.9408) knots 0 0 0 0 1 1 1 1
  spline S40 degree 3 poles (4.7428, -34.8996) (4.7662, -34.8763) (4.5158, -34.5393) (4.1864, -34.1508) knots 0 0 0 0 1 1 1 1
  line L236 (1.5985, -34.229) -> (0.018, -34.2481)
  line L237 (15.6741, -31.3696) -> (16.0298, -31.405)
  line L238 (14.8076, -30.0066) -> (14.8539, -30.0528)
  line L239 (17.9809, -36.1297) -> (17.9809, -36.6579)
  line L240 (-6.1799, -35.2972) -> (-4.5105, -35.2972)
  line L241 (14.9001, -30.099) -> (15.1093, -30.7166)
  line L242 (14.5963, -38.174) -> (14.4029, -37.8789)
  line L243 (12.2729, -35.8435) -> (12.2729, -36.2659)
  line L244 (15.1809, -36.6493) -> (15.0533, -37.2838)
  line L245 (16.8062, -34.3595) -> (17.3935, -34.9805)
  line L246 (14.813, -37.6718) -> (14.8986, -37.6701)
  line L247 (14.9692, -37.4199) -> (14.8851, -37.5559)
  line L248 (16.1543, -36.1377) -> (16.1543, -35.3811)
  line L249 (12.0608, -36.4714) -> (11.9832, -36.1575)
  line L250 (15.7316, -33.9011) -> (14.8415, -33.8993)
  line L251 (16.1543, -34.6244) -> (16.4451, -34.4919)
  line L252 (12.3904, -30.4718) -> (12.5111, -30.2464)
  line L253 (16.4451, -34.4919) -> (16.7359, -34.3595)
  line L254 (19.3088, -35.8401) -> (19.1252, -35.8401)
  line L255 (12.1669, -36.5799) -> (12.0608, -36.4714)
  line L256 (12.2135, -31.1869) -> (12.2698, -30.6972)
  line L257 (1.5985, -36.3969) -> (1.5985, -34.229)
  spline S41 degree 3 poles (4.6394, -32.3731) (3.6867, -32.3998) (3.5037, -32.372) (3.3016, -32.1699) knots 0 0 0 0 1 1 1 1
  line L258 (13.5266, -36.8009) -> (13.4862, -36.3507)
  line L259 (12.2268, -32.6471) -> (12.8259, -33.0665)
  line L260 (19.5732, -35.6152) -> (19.2864, -35.6152)
  line L261 (-4.5105, -36.4338) -> (-6.0733, -36.4338)
  line L262 (16.1543, -35.3811) -> (16.1543, -34.6244)
  line L263 (14.7897, -38.4692) -> (14.5963, -38.174)
  spline S42 degree 3 poles (6.7591, -38.5648) (4.4191, -38.5648) (4.387, -38.5629) (4.1551, -38.405) knots 0 0 0 0 1 1 1 1
  line L264 (12.2698, -30.6972) -> (12.3904, -30.4718)
  line L265 (16.4741, -30.0061) -> (17.1419, -29.8466)
  spline S43 degree 3 poles (4.4993, -34.942) (4.6099, -34.942) (4.7195, -34.923) (4.7428, -34.8996) knots 0 0 0 0 1 1 1 1
  line L266 (12.2729, -36.6883) -> (12.1669, -36.5799)
  line L267 (11.8521, -32.8666) -> (12.0877, -32.6471)
  line L268 (17.3935, -34.9805) -> (17.9809, -35.6015)
  line L269 (14.2584, -37.5559) -> (13.8925, -37.1784)
  line L270 (14.8441, -38.4692) -> (14.7897, -38.4692)
  line L271 (15.3185, -31.3343) -> (15.6741, -31.3696)
  line L272 (14.8851, -37.5559) -> (14.5718, -37.5559)
  line L273 (15.3086, -36.0148) -> (15.1809, -36.6493)
  spline S44 degree 3 poles (-2.1671, -33.255) (-1.9378, -33.0989) (-1.8867, -33.0951) (-0.007, -33.0952) knots 0 0 0 0 1 1 1 1
  spline S45 degree 3 poles (4.1864, -34.1508) (3.7893, -33.6823) (3.5875, -33.3855) (3.5875, -33.2697) knots 0 0 0 0 1 1 1 1
  line L274 (2.7351, -36.1957) -> (2.7351, -38.5648)
  line L275 (0.018, -34.2481) -> (-1.5626, -34.2672)
  line L276 (2.7351, -38.5648) -> (2.1668, -38.5648)
  spline S46 degree 3 poles (3.5875, -33.2697) (3.5875, -33.0975) (3.5961, -33.0951) (4.212, -33.0951) knots 0 0 0 0 1 1 1 1
  line L277 (12.0893, -35.8435) -> (12.2729, -35.8435)
  line L278 (13.6805, -35.444) -> (14.0854, -34.9588)
  line L279 (13.4458, -35.9006) -> (13.5631, -35.6723)
  line L280 (14.5, -41.5) -> (-14.5, -41.5)
  line L281 (15, -27.5) -> (-15, -27.5)
  line L282 (0, -42.5744) -> (0, -26.4256)
  line L283 (0, -34.5) -> (0.323, -34.5)
  spline S47 degree 3 poles (-6.2792, -33.0952) (-4.4394, -33.095) (-4.3839, -33.0991) (-4.1558, -33.2542) knots 0 0 0 0 0.998349 0.998349 0.998349 0.998349
  line L284 (-4.1546, -33.255) -> (-4.1558, -33.2542)
  constraint coincident L131.start L158.end
  constraint midpoint L282 L283.start
emboss "Gravure en relief3" depth 0.3 profiles "Esquisse9" section 1 onto face at (14.9255, -36.5, -101.4935) on bodies 7 bodies 7
pattern_circular "Réseau C1" count 3 over 360 about axis through (0, -41, -100) along (0, 1, 0) of "Gravure en relief3"
sketch "Esquisse10" plane through (0, -27.5, 0) normal (0, 1, 0) x (-1, 0, 0)
  circle A0 centre (0, -100) radius 15
  circle A1 centre (0, -100) radius 4.75
  dimension "d121" = 9.5
  constraint concentric A0 A1
  measures "d121" diameter of A1
extrude "Extrusion20" cut sketch "Esquisse10" against normal blind 8.5 contours A1 bodies 7
chamfer "Chanfrein2" distance 0.5 angle 45 1 edges at (-13.9849, -27.5, -94.5758) on bodies 7
fillet "Congé9" radius 0.5 1 edges at (4.4286, -27.5, -98.2823) on bodies 7
hidden bodies 1 2 5 6
